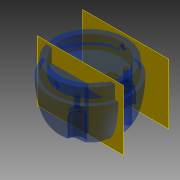
# Autodesk Inventor part: Handle_2_Back
Saved by Autodesk Inventor 2011 SP2 (Build 150309200, 309)
## iProperties
Created: 2012-03-19
Part Number: Handle_2_Back
Document SubType Name: Modeling
Designer: sungwook
Density: 1 g/cm^3
Author: sungwook
Autodesk Inventor part; units mm, degrees
ref_plane "YZ Plane" through (0, 0, 0) normal (1, 0, 0) x (0, 1, 0)
ref_plane "XY Plane" through (0, 0, 0) normal (0, 0, 1) x (1, 0, 0)
sketch "Sketch1" plane through (0, 0, 0) normal (0, 0, 1) x (1, 0, 0)
  point P0 (0, 0)
sketch "Sketch2" plane through (0, 0, 0) normal (1, 0, 0) x (0, 1, 0)
  line L0 (-13.0429, 0) -> (13.0429, 0)
  line L1 (13.0429, 0) -> (13.0429, 3.3095)
  line L2 (13.0429, 3.3095) -> (-13.0429, 3.3095)
  line L3 (-13.0429, 3.3095) -> (-13.0429, 0)
  line L4 (0, 0) -> (0, -15)
  line L5 (0, -15) -> (-8, -15)
  line L6 (-14.2875, 0) -> (14.2875, 0)
  line L7 (14.2875, 0) -> (14.2875, 6.8547)
  line L8 (14.2875, 6.8547) -> (-14.2875, 6.8547)
  line L9 (-14.2875, 6.8547) -> (-14.2875, 0)
  spline S0 degree 4 poles (-14.2875, 0) (-14.2875, -4.9566) (-13.3423, -10.7623) (-11.8115, -15) (-8, -15) knots 0 0 0 0 0 1 1 1 1 1
  point P0 (-12.3627, -11.4481)
  dimension "d1" = 26.0858
  dimension "d2" = 8
  dimension "d3" = 15
  dimension "d4" = 28.575
  constraints: 20 end point, 5 parallel, 3 coincident, 3 horizontal, 3 perpendicular, 2 midpoint, 1 point on line, 1 vertical, 3 other
  measures "d1" distance of L0.end L0.start
  measures "d2" distance of L4.end L5.end
  measures "d3" distance between parallel lines of L5 L0
  measures "d4" distance between parallel lines of L7 L9
revolve "Revolution1" add sketch "Sketch2" angle 360 about axis through (0, 0, 0) along (0, 0, -1) contours L0 L4 L5 S0 L6
sketch "Sketch3" plane through (0, 0, 0) normal (0, 0, 1) x (1, 0, 0)
  circle A0 centre (0, 0) radius 14.2875 projected
  circle A1 centre (0, 0) radius 13.0429
  circle A2 centre (0, 0) radius 11
  point P0 (0, -14.2875)
  dimension "d6" = 26.0858
  dimension "d7" = 22
  constraints: 2 centre point, 2 coincident, 1 vertical alignment
  measures "d6" diameter of A1
  measures "d7" diameter of A2
extrude "Extrusion1" add sketch "Sketch3" along normal blind 5 contours A1
hole "Hole1" at (0, 0, 0) direction (0, 0, -1) diameter 3 end through all
sketch "Sketch6" plane through (0, 0, 0) normal (0, 0, 1) x (1, 0, 0)
  circle A0 centre (0, 0) radius 12
  point P0 (4.074, -8.737)
  point P1 (4.82, 8.349)
  point P2 (-9.494, -1.674)
  dimension "d22" = -8.737
  dimension "d23" = 8.349
  dimension "d24" = 1.674
  dimension "d25" = 4.074
  dimension "d26" = 4.82
  constraints: 1 centre point, 1 coincident
  measures "d22" vertical distance of point (0, 0) point (4.074, -8.737)
  measures "d23" vertical distance of point (0, 0) point (4.82, 8.349)
  measures "d24" vertical distance of point (0, 0) point (-9.494, -1.674)
  measures "d25" horizontal distance of point (4.074, -8.737) point (0, 0)
  measures "d26" horizontal distance of point (0, 0) point (4.82, 8.349)
hole "Hole2" at (-9.494, -1.674, 0) at (4.82, 8.349, 0) at (4.074, -8.737, 0) direction (0, 0, -1) diameter 1.7 end through all clearance for "Flat Head Machine Screw (82)" size "#0" standard "Ansi Unified Screw Threads"
sketch "Sketch8" plane through (0, 0, 0) normal (0, 1, 0) x (-1, 0, 0)
  point P0 (0, 0)
sketch "Sketch9" plane through (0, 0, -15) normal (0, 0, -1) x (-1, 0, 0)
  circle A0 centre (0, 0) radius 1.5 projected
  line L0 (-10.3562, 5) -> (-3, 5)
  line L1 (-3, 5) -> (-3, -5)
  line L2 (-3, -5) -> (-10.3562, -5)
  line L3 (20.0025, 0) -> (-20.0025, 0) projected
  line L4 (0, -20.0025) -> (0, 20.0025) projected
  circle A1 centre (-4.82, 8.349) radius 0.85 projected
  circle A2 centre (-4.074, -8.737) radius 0.85 projected
  circle A3 centre (0, 0) radius 8 projected
  arc A4 (-10.3562, 5) -> (-10.3562, -5) centre (0, 0) ccw
  point P0 (0, -8)
  point P1 (-10.7619, 0)
  dimension "d34" = 3
  dimension "d35" = 8.349
  dimension "d36" = 8.737
  dimension "d37" = 10
  constraints: 6 end point, 2 point on circle, 1 centre point, 1 coincident, 1 horizontal, 1 horizontal alignment, 1 parallel, 1 perpendicular, 1 vertical alignment
  measures "d34" distance between parallel lines of L4 L1
  measures "d35" vertical distance of A0.centre A1.centre
  measures "d36" vertical distance of A2.centre A0.centre
  measures "d37" distance between parallel lines of L2 L0
extrude "Extrusion2" cut sketch "Sketch9" against normal through all contours L3 A3 L0 L1 | L1 L2 A3 L3 | A3 L3 A4 L0 | L2 A4 L3 A3
sketch "Sketch10" plane through (6.245, 5, -15) normal (0, 0, -1) x (-1, 0, 0)
  arc A0 (2.1327, 3.8197) -> (2.1327, 3.8197) centre (2.1327, 3.8197) ccw projected
  arc A1 (3.0175, -13.6604) -> (3.0175, -13.6604) centre (3.0175, -13.6604) ccw projected
  arc A2 (16.4746, -6.2481) -> (16.4746, -6.2481) centre (16.4746, -6.2481) ccw projected
  circle A3 centre (1.425, 3.349) radius 0.85 projected
  circle A4 centre (2.171, -13.737) radius 2.5
  circle A5 centre (2.171, -13.737) radius 0.85 projected
  circle A6 centre (15.739, -6.674) radius 2.5
  circle A7 centre (15.739, -6.674) radius 0.85 projected
  circle A8 centre (1.425, 3.349) radius 2.5
  dimension "d43" = 5
  dimension "d44" = 5
  dimension "d59" = 5
  constraints: 3 centre point, 1 coincident, 8 other
  measures "d43" diameter of A6
  measures "d44" diameter of A4
  measures "d59" diameter of A8
ref_plane "Work Plane1" through (6.245, 5, -17) normal (0, 0, -1) x (-1, 0, 0)
sketch "Sketch11" plane through (6.245, 5, -17) normal (0, 0, -1) x (-1, 0, 0)
  arc A0 (2.1327, 3.8197) -> (2.1327, 3.8197) centre (2.1327, 3.8197) ccw projected
  arc A1 (16.4746, -6.2481) -> (16.4746, -6.2481) centre (16.4746, -6.2481) ccw projected
  arc A2 (3.0175, -13.6604) -> (3.0175, -13.6604) centre (3.0175, -13.6604) ccw projected
  circle A3 centre (1.425, 3.349) radius 2.5
  circle A4 centre (1.425, 3.349) radius 0.85 projected
  circle A5 centre (2.171, -13.737) radius 2.5
  circle A6 centre (15.739, -6.674) radius 2.5
  circle A7 centre (15.739, -6.674) radius 0.85 projected
  circle A8 centre (2.171, -13.737) radius 0.85 projected
  point P0 (6.245, -5)
  dimension "d61" = 5
  dimension "d62" = 5
  dimension "d63" = 5
  constraints: 3 centre point, 9 other
  measures "d61" diameter of A3
  measures "d62" diameter of A5
  measures "d63" diameter of A6
hole "Hole5" at (4.82, 8.349, -17) at (-9.494, -1.674, -17) at (4.074, -8.737, -17) direction (0, 0, 1) diameter 5 depth 10
sketch "Sketch12" plane through (-9.494, -1.674, -7) normal (0, 0, -1) x (-1, 0, 0)
  circle A0 centre (0, 0) radius 0.85 projected
  circle A1 centre (-14.314, 10.023) radius 0.85 projected
  circle A2 centre (-13.568, -7.063) radius 0.85 projected
  line L0 (-12.264, 8.8394) -> (-14.3141, 7.6559)
  line L1 (-14.3141, 7.6559) -> (-16.364, 8.8395)
  line L2 (-16.364, 8.8395) -> (-16.364, 11.2066)
  line L3 (-16.364, 11.2066) -> (-14.3139, 12.3901)
  line L4 (-14.3139, 12.3901) -> (-12.264, 11.2065)
  line L5 (-12.264, 11.2065) -> (-12.264, 8.8394)
  line L6 (-0.411, -2.3312) -> (-2.2244, -0.8096)
  line L7 (-2.2244, -0.8096) -> (-1.8133, 1.5216)
  line L8 (-1.8133, 1.5216) -> (0.411, 2.3312)
  line L9 (0.411, 2.3312) -> (2.2244, 0.8096)
  line L10 (2.2244, 0.8096) -> (1.8133, -1.5216)
  line L11 (1.8133, -1.5216) -> (-0.411, -2.3312)
  line L12 (-9.494, 1.674) -> (-14.314, 10.023)
  line L13 (-9.494, 1.674) -> (0, 0)
  line L14 (-9.494, 1.674) -> (-13.568, -7.063)
  line L15 (-11.4226, -8.0634) -> (-13.3617, -9.4211)
  line L16 (-13.3617, -9.4211) -> (-15.507, -8.4208)
  line L17 (-15.507, -8.4208) -> (-15.7134, -6.0626)
  line L18 (-15.7134, -6.0626) -> (-13.7743, -4.7049)
  line L19 (-13.7743, -4.7049) -> (-11.629, -5.7052)
  line L20 (-11.629, -5.7052) -> (-11.4226, -8.0634)
  dimension "d71" = 4.1
  dimension "d72" = 4.1
  dimension "d73" = 4.1
  constraints: 42 end point, 3 coincident, 3 perpendicular, 40 other
  measures "d71" distance between parallel lines of L16 L19
  measures "d72" distance between parallel lines of L4 L1
  measures "d73" distance between parallel lines of L6 L9
extrude "Extrusion3" cut sketch "Sketch12" against normal blind 2 contours L7 L8 L9 L10 L11 L6 | A2 | L19 L20 L15 L16 L17 L18 | L0 L1 L2 L3 L4 L5
ref_plane "Work Plane2" through (0, 13.0429, 0) normal (0, 1, 0) x (-1, 0, 0)
sketch "Sketch13" plane through (0, 13.0429, 0) normal (0, 1, 0) x (-1, 0, 0)
  line L0 (-13.0429, 5) -> (13.0429, 5) projected
  line L1 (-13.0429, 0) -> (13.0429, 0) projected
  line L2 (0, -19.0003) -> (0, 9.0001) projected
  point P0 (0, 0)
  point P1 (0, 2.5)
  dimension "d76" = 2.5
  constraints: 1 point on line
  measures "d76" distance from line of point (0, 2.5) L0
hole "Hole6" at (0, 13.0429, 2.5) direction (0, -1, 0) diameter 1.694 end through all thread size "2-56 UNC" class "2B" standard "ANSI Unified Screw Threads"
ref_plane "Work Plane3" through (0, -3.5, 0) normal (0, 1, 0) x (-1, 0, 0)
body "Solid1"
